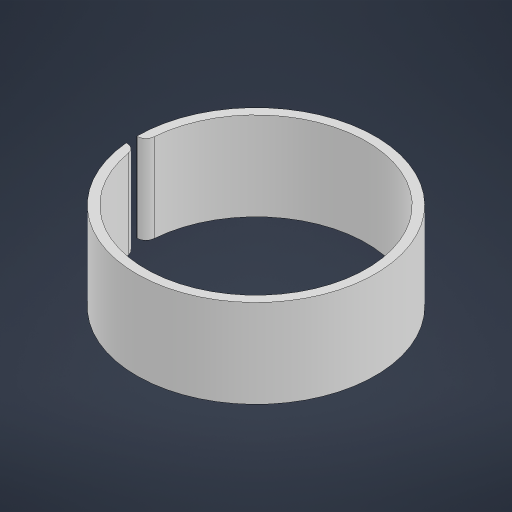
# Autodesk Inventor part: Senban_zigu2
Saved by Autodesk Inventor 2024.2 (Build 282272000, 272)
## iProperties
Created: 2024-02-19
Part Number: Senban_zigu2
Material: 一般
Document SubType Name: Modeling
Designer: Hanaoka
Density: 1 g/cm^3
Appearance: 既定
Author: Hanaoka
Autodesk Inventor part; units mm, degrees
ref_plane "YZ Plane" through (0, 0, 0) normal (1, 0, 0) x (0, 1, 0)
ref_plane "XZ Plane" through (0, 0, 0) normal (0, 1, 0) x (-1, 0, 0)
ref_plane "XY Plane" through (0, 0, 0) normal (0, 0, 1) x (1, 0, 0)
sketch "スケッチ1" plane through (0, 0, 0) normal (0, 1, 0) x (-1, 0, 0)
  arc A0 (26.9342, 2.5) -> (27.05, 0) centre (0, 0) ccw
  arc A1 (24.9249, 2.5) -> (25.05, 0) centre (0, 0) ccw
  line L0 (26.9342, 2.5) -> (24.9249, 2.5)
  line L1 (39.5466, 0) -> (-39.5755, 0) projected
  dimension "d0" = 25.05
  dimension "d1" = 2
  dimension "d2" = 2.5
  constraints: 4 point on circle, 2 centre point, 2 coincident, 2 end point, 1 parallel
  measures "d0" radius of A1
  measures "d1" radial gap between concentric circles of A0 A1
  measures "d2" distance between parallel lines of L1 L0
extrude "押し出し1" add sketch "スケッチ1" along normal blind 20 contours L0 A1 L1 A0 | L1 A1 A0
fillet "フィレット1" radius 2 2 edges at (-25.05, 10, 0) (-24.9249, 10, 2.5)
